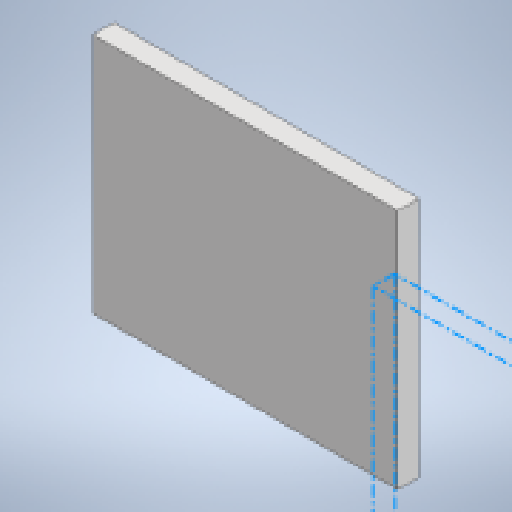
# Autodesk Inventor part: couvercle
Saved by Autodesk Inventor 2024 (Build 280153000, 153)
## iProperties
Created: 2024-03-05
Part Number: couvercle
Material: Générique
Document SubType Name: Modeling
Designer: phaly
Density: 1 g/cm^3
Appearance: Par défaut
Author: phaly
Autodesk Inventor part; units mm, degrees
ref_plane "YZ Plane" through (0, 0, 0) normal (1, 0, 0) x (0, 1, 0)
ref_plane "XZ Plane" through (0, 0, 0) normal (0, 1, 0) x (-1, 0, 0)
sketch "Esquisse1" plane through (0, 0, 0) normal (0, 0, 1) x (1, 0, 0)
  line L0 (-45.5759, 93.3928) -> (-189.5759, 93.3928) projected
  line L1 (-189.5759, 93.3928) -> (-189.5759, -20.6072) projected
  line L2 (-45.5759, -20.6072) -> (-45.5759, 93.3928) projected
  line L3 (-189.5759, -20.6072) -> (-45.5759, -20.6072) projected
  line L4 (-189.5759, 93.3928) -> (-45.5759, 93.3928)
  line L5 (-45.5759, 93.3928) -> (-45.5759, -20.6072)
  line L6 (-45.5759, -20.6072) -> (-189.5759, -20.6072)
  line L7 (-189.5759, -20.6072) -> (-189.5759, 93.3928)
  point P0 (0, 0)
  constraints: 8 end point, 2 parallel, 1 horizontal, 1 perpendicular
extrude "Extrusion1" add sketch "Esquisse1" along normal blind 21
sketch "Esquisse2" plane through (0, 0, 0) normal (0, 0, -1) x (-1, 0, 0)
  line L0 (186.5759, -17.6072) -> (48.5759, -17.6072)
  line L1 (48.5759, -17.6072) -> (48.5759, 90.3928)
  line L2 (48.5759, 90.3928) -> (186.5759, 90.3928)
  line L3 (186.5759, 90.3928) -> (186.5759, -17.6072)
  line L4 (189.5759, -20.6072) -> (45.5759, -20.6072) projected
  line L5 (45.5759, 93.3928) -> (189.5759, 93.3928) projected
  line L6 (189.5759, 93.3928) -> (189.5759, -20.6072) projected
  line L7 (45.5759, -20.6072) -> (45.5759, 93.3928) projected
  point P0 (0, 0)
  dimension "d2" = 3
  dimension "d4" = 3
  dimension "d5" = 3
  dimension "d6" = 3
  constraints: 8 end point, 2 parallel, 1 horizontal, 1 perpendicular
  measures "d2" distance between parallel lines of L4 L0
  measures "d4" distance between parallel lines of L6 L3
  measures "d5" distance between parallel lines of L5 L2
  measures "d6" distance between parallel lines of L7 L1
extrude "Extrusion3" cut sketch "Esquisse2" against normal blind 17 contours L0 L1 L2 L3
sketch "Esquisse3" plane through (-45.5759, -20.6072, 0) normal (1, 0, 0) x (0, 0, -1)
  line L0 (-15, 47.25) -> (0, 47.25)
  line L1 (0, 47.25) -> (0, 91.25)
  line L2 (0, 91.25) -> (-15, 91.25)
  line L3 (-15, 91.25) -> (-15, 47.25)
  line L4 (0, -22.8) -> (0, 136.8) projected
  line L5 (0, 0) -> (-21, 0) projected
  point P0 (0, 20.6072)
  point P1 (-10.5, -7.9486)
  point P2 (-10.5, 0)
  dimension "d11" = 15
  dimension "d12" = 44
  dimension "d19" = 47.25
  constraints: 8 end point, 2 parallel, 1 collinear, 1 horizontal, 1 midpoint, 1 perpendicular
  measures "d11" distance of L0.start L0.end
  measures "d12" distance of L2.end L0.start
  measures "d19" distance from line of point (-10.5, 0) L0
ref_plane "Plan de construction1" through (-50.5759, 25.8928, -3.5) normal (-1, 0, 0) x (0, 0, 1)
extrude "Extrusion4" cut sketch "Esquisse3" against normal up to surface (5 mm away)
equation "\"d4\" = d2"
equation "\"d5\" = d2"
equation "\"d6\" = d4"
